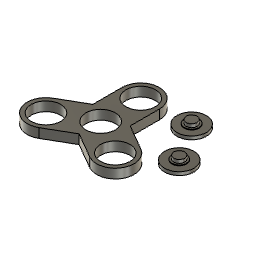
fidget spinner v1 (Autodesk Fusion 360 design; units mm, degrees)
Autodesk Fusion 360 part; units mm, degrees
sketch "Sketch1" plane through (0, 0, 0) normal (0, 0, 1) x (1, 0, 0)
  line L0 (30, -30) -> (2, -30)
  line L1 (2, -30) -> (2, 0)
  line L2 (2, 0) -> (30, 0)
  line L3 (30, 0) -> (30, -30)
  circle A0 centre (16, -30) radius 14
  circle A1 centre (16, -30) radius 11.025
  circle A2 centre (16, 0) radius 14
  circle A3 centre (16, 0) radius 11.025
  dimension "d1" = 28
  dimension "d2" = 30
  dimension "d3" = 28
  dimension "d4" = 22.05
  dimension "d5" = 28
  dimension "d6" = 22.05
  constraint horizontal L0
  constraint vertical L1
  constraint horizontal L2
  constraint vertical L3
  constraint midpoint L0 A0.centre
  constraint concentric A0 A1
  constraint midpoint L2 A2.centre
  constraint concentric A2 A3
  measures "d1" distance of L0.start L0.end
  measures "d2" distance of L0.start L2.end
  measures "d3" diameter of A0
  measures "d4" diameter of A1
  measures "d5" diameter of A2
  measures "d6" diameter of A3
extrude "Extrude1" add sketch "Sketch1" along normal blind 7 contours L0 A0 A1 | L1 L3 A0 A2 | L0 A0 A1 | L2 A2 A3 | L2 A2 A3 makes body 1
pattern_circular "C-Pattern1" count 3 over 360 about axis through (16, -30, 0) along (0, 0, 1) of bodies 1 makes body 2 at (-6.2618, -28.2524, 0) makes body 3 at (32.3633, -24.8469, 0)
combine "Combine1" operation add target body 1 tool bodies 2 3
sketch "Sketch2" plane through (0, 0, 0) normal (0, 0, 1) x (1, 0, 0)
  circle A0 centre (85, -5) radius 11
  circle A1 centre (85, -5) radius 5.5
  circle A2 centre (85, -5) radius 4.075
  dimension "d11" = 22
  dimension "d12" = 11
  dimension "d13" = 8.15
  constraint concentric A0 A1
  constraint concentric A0 A2
  measures "d11" diameter of A0
  measures "d12" diameter of A1
  measures "d13" diameter of A2
extrude "Extrude2" add sketch "Sketch2" along normal blind 2.5 separate body contours A0 makes body 4
extrude "Extrude3" add sketch "Sketch2" along normal blind 3 contours A1 bodies 4
extrude "Extrude4" add sketch "Sketch2" along normal blind 5.5 contours A2 bodies 4
copy_body "CopyPasteBodies1" bodies 4 makes body 5
move_body "Move1" bodies 5 to x (1, 0, 0) y (0, 1, 0) z (0, 0, 1) at (0, 50, 0)
move_body "Move2" bodies 5 to x (1, 0, 0) y (0, 1, 0) z (0, 0, 1) at (-37.8531, -37.9872, -0.1343)
move_body "Move3" bodies 4 to x (1, 0, 0) y (0, 1, 0) z (0, 0, 1) at (-18.1015, -17.027, 1.0745)
